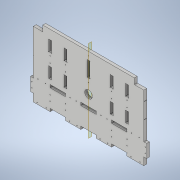
# Autodesk Inventor part: Side_one
Saved by Autodesk Inventor 2020 (Build 240168000, 168)
## iProperties
Created: 2019-12-17
Part Number: Side_one
Material: Generic
Document SubType Name: Modeling
Designer: fabfarm
Density: 1 g/cm^3
Appearance: Default
Author: fabfarm
Autodesk Inventor part; units mm, degrees
ref_plane "YZ Plane" through (0, 0, 0) normal (1, 0, 0) x (0, 1, 0)
ref_plane "XZ Plane" through (0, 0, 0) normal (0, 1, 0) x (-1, 0, 0)
ref_plane "XY Plane" through (0, 0, 0) normal (0, 0, 1) x (1, 0, 0)
sketch "Sketch1" plane through (0, 0, 0) normal (0, 0, 1) x (1, 0, 0)
  line L0 (0, 0) -> (-756, 0)
  line L1 (-756, 0) -> (-756, 464.3)
  line L2 (-756, 464.3) -> (0, 464.3)
  line L3 (0, 464.3) -> (0, 0)
  dimension "d0" = 464.3
  dimension "d1" = 756
  constraints: 8 end point, 2 parallel, 1 horizontal, 1 perpendicular
  measures "d0" distance of L2.end L0.start
  measures "d1" distance of L0.start L0.end
extrude "Extrusion1" add sketch "Sketch1" along normal blind 18.55
sketch "Sketch2" plane through (0, 0, 18.55) normal (0, 0, 1) x (1, 0, 0)
  line L0 (-756, 464.3) -> (-756, 0) projected
  line L1 (-756, 464.3) -> (-737.45, 464.3)
  line L2 (-737.45, 464.3) -> (-737.45, 359.9)
  line L3 (-737.45, 359.9) -> (-756, 359.9)
  line L4 (-756, 359.9) -> (-756, 464.3)
  line L5 (0, 464.3) -> (-756, 464.3) projected
  line L6 (-756, 259.9) -> (-737.45, 259.9)
  line L7 (-737.45, 259.9) -> (-737.45, 134.8)
  line L8 (-737.45, 134.8) -> (-756, 134.8)
  line L9 (-756, 134.8) -> (-756, 259.9)
  point P0 (-756, 359.9)
  point P1 (-756, 134.8)
  dimension "d54" = 18.55
  dimension "d55" = 104.4
  dimension "d86" = 100
  dimension "d87" = 125.1
  constraints: 16 end point, 4 parallel, 2 collinear, 2 horizontal, 2 perpendicular, 2 point on line
  measures "d54" distance of L1.start L1.end
  measures "d55" distance of L1.end L2.end
  measures "d86" distance between parallel lines of L6 L3
  measures "d87" distance of L6.end L7.end
extrude "Extrusion2" cut sketch "Sketch2" against normal blind 18.55
ref_plane "Work Plane1" through (-378, 259.9, 0) normal (-1, 0, 0) x (0, 0, 1)
mirror "Mirror1" about plane through (-378, 259.9, 0) normal (-1, 0, 0) of "Extrusion2"
sketch "Sketch3" plane through (0, 0, 18.55) normal (0, 0, 1) x (1, 0, 0)
  line L0 (0, 464.3) -> (-756, 464.3) projected
  line L1 (-756, 426.35) -> (-676, 426.35)
  line L2 (-676, 426.35) -> (-676, 464.3)
  line L3 (-676, 464.3) -> (-756, 464.3)
  line L4 (-756, 464.3) -> (-756, 426.35)
  point P0 (0, 0)
  point P1 (-18.55, 350)
  point P2 (0, 464.3)
  dimension "d19" = 80
  dimension "d22" = 37.95
  constraints: 8 end point, 2 perpendicular, 1 parallel, 2 other
  measures "d19" distance of L3.end L2.end
  measures "d22" distance of L3.end L1.start
extrude "Extrusion3" cut sketch "Sketch3" against normal blind 18.55
mirror "Mirror2" about plane through (-378, 259.9, 0) normal (-1, 0, 0) of "Extrusion3"
sketch "Sketch4" plane through (0, 0, 18.55) normal (0, 0, 1) x (1, 0, 0)
  line L0 (-628, 134.8) -> (-528, 134.8)
  line L1 (-528, 134.8) -> (-528, 153.35)
  line L2 (-528, 153.35) -> (-628, 153.35)
  line L3 (-628, 153.35) -> (-628, 134.8)
  line L4 (-428, 134.8) -> (-328, 134.8)
  line L5 (-328, 134.8) -> (-328, 153.35)
  line L6 (-328, 153.35) -> (-428, 153.35)
  line L7 (-428, 153.35) -> (-428, 134.8)
  line L8 (-228, 134.8) -> (-128, 134.8)
  line L9 (-128, 134.8) -> (-128, 153.35)
  line L10 (-128, 153.35) -> (-228, 153.35)
  line L11 (-228, 153.35) -> (-228, 134.8)
  line L12 (0, 0) -> (0, 359.9) projected
  line L13 (-756, 359.9) -> (-756, 0) projected
  line L14 (-737.45, 134.8) -> (-756, 134.8) projected
  line L15 (-756, 259.9) -> (-737.45, 259.9) projected
  line L16 (-80, 464.3) -> (-676, 464.3) projected
  line L17 (-378, 464.3) -> (-378, 153.35) construction
  dimension "d59" = 100
  dimension "d60" = 100
  dimension "d61" = 100
  dimension "d62" = 100
  dimension "d63" = 100
  dimension "d66" = 18.55
  constraints: 26 end point, 6 parallel, 5 collinear, 3 horizontal, 3 perpendicular, 2 midpoint, 1 vertical
  measures "d59" distance of L1.end L2.end
  measures "d60" distance of L5.end L6.end
  measures "d61" distance between parallel lines of L1 L7
  measures "d62" distance between parallel lines of L11 L5
  measures "d63" distance of L9.end L10.end
  measures "d66" distance of L2.end L0.start
extrude "Extrusion4" cut sketch "Sketch4" against normal blind 20
sketch "Sketch6" plane through (0, 0, 18.55) normal (0, 0, 1) x (1, 0, 0)
  line L0 (-328, 400.4) -> (-428, 400.4)
  line L1 (-428, 400.4) -> (-428, 425.4)
  line L2 (-428, 425.4) -> (-328, 425.4)
  line L3 (-328, 425.4) -> (-328, 400.4)
  line L4 (-328, 400.4) -> (-428, 425.4) construction
  line L5 (-428, 400.4) -> (-328, 425.4) construction
  line L6 (-378, -92.86) -> (-378, 557.16) projected
  line L7 (-80, 464.3) -> (-676, 464.3) projected
  point P0 (0, 0)
  point P1 (-378, 412.9)
  dimension "d38" = 25
  dimension "d39" = 100
  dimension "d40" = 38.9
  constraints: 12 end point, 2 midpoint, 2 parallel, 1 horizontal, 1 perpendicular, 1 point on line
  measures "d38" distance of L0.end L1.end
  measures "d39" distance of L1.end L2.end
  measures "d40" distance between parallel lines of L7 L2
extrude "Extrusion6" [suppressed]
fillet "Fillet1" [suppressed]
sketch "Sketch7" plane through (0, 0, 18.55) normal (0, 0, 1) x (1, 0, 0)
  line L0 (-637.45, 183.35) -> (-618.9, 183.35)
  line L1 (-618.9, 183.35) -> (-618.9, 253.85)
  line L2 (-618.9, 253.85) -> (-637.45, 253.85)
  line L3 (-637.45, 253.85) -> (-637.45, 183.35)
  line L4 (-537.5, 183.35) -> (-518.95, 183.35)
  line L5 (-518.95, 183.35) -> (-518.95, 253.85)
  line L6 (-518.95, 253.85) -> (-537.5, 253.85)
  line L7 (-537.5, 253.85) -> (-537.5, 183.35)
  line L8 (-676, 464.3) -> (-676, 426.35) projected
  line L9 (-628, 153.35) -> (-528, 153.35) projected
  line L10 (-737.45, 259.9) -> (-737.45, 134.8) projected
  point P0 (0, 0)
  dimension "d44" = 81.4
  dimension "d45" = 18.55
  dimension "d46" = 70.5
  dimension "d72" = 30
  dimension "d194" = 100
  constraints: 16 end point, 4 parallel, 2 horizontal, 2 perpendicular, 2 point on line, 1 collinear
  measures "d44" distance between parallel lines of L7 L1
  measures "d45" distance of L1.end L2.end
  measures "d46" distance of L2.end L0.start
  measures "d72" distance between parallel lines of L9 L0
  measures "d194" distance between parallel lines of L10 L3
extrude "Extrusion7" cut sketch "Sketch7" against normal blind 20
mirror "Mirror3" about plane through (-378, 259.9, 0) normal (-1, 0, 0) of "Extrusion7"
sketch "Esquisse8" plane through (0, 0, 0) normal (0, 0, -1) x (-1, 0, 0)
  line L0 (137.1, 334.35) -> (118.55, 334.35)
  line L1 (118.55, 334.35) -> (118.55, 404.85)
  line L2 (118.55, 404.85) -> (137.1, 404.85)
  line L3 (137.1, 404.85) -> (137.1, 334.35)
  line L4 (218.5, 404.85) -> (237.05, 404.85)
  line L5 (237.05, 404.85) -> (237.05, 334.35)
  line L6 (237.05, 334.35) -> (218.5, 334.35)
  line L7 (218.5, 334.35) -> (218.5, 404.85)
  line L8 (118.55, 183.35) -> (118.55, 253.85) projected
  line L9 (137.1, 253.85) -> (137.1, 183.35) projected
  line L10 (218.5, 183.35) -> (218.5, 253.85) projected
  line L11 (237.05, 253.85) -> (237.05, 183.35) projected
  line L12 (137.1, 253.85) -> (118.55, 253.85) projected
  point P0 (0, 0)
  dimension "d51" = 70.5
  dimension "d90" = 80.5
  constraints: 16 end point, 4 collinear, 4 parallel, 2 horizontal, 2 perpendicular, 2 point on line
  measures "d51" distance of L0.end L1.end
  measures "d90" distance between parallel lines of L0 L12
extrude "Extrusion8" cut sketch "Esquisse8" against normal blind 20
mirror "Symétrie4" about plane through (-378, 259.9, 0) normal (-1, 0, 0) of "Extrusion8"
sketch "Esquisse9" plane through (0, 0, 18.55) normal (0, 0, 1) x (1, 0, 0)
  circle A0 centre (-738.5708, 361.0208) radius 1.585
  circle A1 centre (-738.5708, 135.9208) radius 1.585
  circle A2 centre (-636.3292, 403.7292) radius 1.585
  circle A3 centre (-638.5708, 333.2292) radius 1.585
  circle A4 centre (-738.5708, 258.7792) radius 1.585
  circle A5 centre (-636.3292, 252.7292) radius 1.585
  circle A6 centre (-620.0208, 252.7292) radius 1.585
  circle A7 centre (-620.0208, 184.4708) radius 1.585
  circle A8 centre (-677.1208, 427.4708) radius 1.585
  circle A9 centre (-626.8792, 152.2292) radius 1.585
  circle A10 centre (-426.8792, 152.2292) radius 1.585
  line L0 (-80, 464.3) -> (-676, 464.3) projected
  line L1 (-378, 464.3) -> (-378, 151.8903) construction
  circle A11 centre (-626.8792, 135.9208) radius 1.585
  circle A12 centre (-426.8792, 135.9208) radius 1.585
  line L2 (-737.45, 359.9) -> (-738.5708, 361.0208) construction
  line L3 (-737.45, 426.35) -> (-737.45, 359.9) projected
  line L4 (-737.45, 259.9) -> (-738.5708, 258.7792) construction
  line L5 (-738.5708, 135.9208) -> (-737.45, 134.8) construction
  line L6 (-737.45, 259.9) -> (-737.45, 134.8) projected
  line L7 (-737.45, 426.35) -> (-676, 426.35) projected
  line L8 (-677.1208, 427.4708) -> (-676, 426.35) construction
  line L9 (-637.45, 404.85) -> (-636.3292, 403.7292) construction
  circle A13 centre (-620.0208, 333.2292) radius 1.585
  line L10 (-620.0208, 333.2292) -> (-618.9, 334.35) construction
  line L11 (-637.45, 334.35) -> (-638.5708, 333.2292) construction
  line L12 (-618.9, 334.35) -> (-637.45, 334.35) projected
  line L13 (-620.0208, 184.4708) -> (-618.9, 183.35) construction
  line L14 (-620.0208, 252.7292) -> (-618.9, 253.85) construction
  line L15 (-618.9, 253.85) -> (-618.9, 183.35) projected
  line L16 (-637.45, 183.35) -> (-636.3292, 184.4708) construction
  line L17 (-618.9, 183.35) -> (-637.45, 183.35) projected
  circle A14 centre (-636.3292, 184.4708) radius 1.585
  line L18 (-618.9, 334.35) -> (-618.9, 464.3) projected
  line L19 (-618.9, 411.8699) -> (-537.5, 369.6) construction
  line L20 (-537.5, 334.35) -> (-537.5, 404.85) construction
  line L21 (-578.2, 390.7349) -> (-579.0419, 153.9249) construction
  circle A15 centre (-519.9798, 403.3156) radius 1.585
  circle A16 centre (-518.2397, 332.8014) radius 1.585
  circle A17 centre (-521.0535, 252.3194) radius 1.585
  circle A18 centre (-537.3616, 252.4354) radius 1.585
  circle A19 centre (-537.8469, 184.1786) radius 1.585
  line L22 (-518.8511, 404.4284) -> (-519.9798, 403.3156) construction
  circle A20 centre (-536.7892, 332.9333) radius 1.585
  line L23 (-536.7892, 332.9333) -> (-537.5, 334.35) construction
  line L24 (-519.3524, 333.9301) -> (-518.2397, 332.8014) construction
  line L25 (-537.8469, 184.1786) -> (-538.9756, 183.0658) construction
  line L26 (-537.3616, 252.4354) -> (-538.4743, 253.5641) construction
  line L27 (-520.4261, 182.934) -> (-521.5389, 184.0627) construction
  circle A21 centre (-521.5389, 184.0627) radius 1.585
  line L28 (-537.5, 334.35) -> (-537.5, 404.85)
  line L29 (-537.3508, 411.5799) -> (-619.0492, 369.8899) construction
  line L30 (-528, 134.8) -> (-628, 134.8) construction
  line L31 (-626.8792, 135.9208) -> (-628, 134.8) construction
  line L32 (-628, 153.35) -> (-528, 153.35) construction
  line L33 (-578, 153.35) -> (-578, 134.8) construction
  circle A22 centre (-529.1208, 152.2292) radius 1.585
  circle A23 centre (-529.1208, 135.9208) radius 1.585
  circle A24 centre (-17.4292, 361.0208) radius 1.585
  circle A25 centre (-17.4292, 135.9208) radius 1.585
  circle A26 centre (-136.0858, 403.632) radius 1.585
  line L34 (-119.6708, 403.7292) -> (-136.0858, 403.632) construction
  circle A27 centre (-119.6708, 403.7292) radius 1.585
  circle A28 centre (-117.4292, 333.2292) radius 1.585
  circle A29 centre (-17.4292, 258.7792) radius 1.585
  circle A30 centre (-119.6708, 252.7292) radius 1.585
  circle A31 centre (-135.9792, 252.7292) radius 1.585
  circle A32 centre (-135.9792, 184.4708) radius 1.585
  circle A33 centre (-78.8792, 427.4708) radius 1.585
  circle A34 centre (-129.1208, 152.2292) radius 1.585
  circle A35 centre (-329.1208, 152.2292) radius 1.585
  circle A36 centre (-129.1208, 135.9208) radius 1.585
  circle A37 centre (-329.1208, 135.9208) radius 1.585
  line L35 (-18.55, 359.9) -> (-17.4292, 361.0208) construction
  line L36 (-18.55, 426.35) -> (-18.55, 359.9)
  line L37 (-18.55, 259.9) -> (-17.4292, 258.7792) construction
  line L38 (-17.4292, 135.9208) -> (-18.55, 134.8) construction
  line L39 (-18.55, 259.9) -> (-18.55, 134.8)
  line L40 (-18.55, 426.35) -> (-80, 426.35)
  line L41 (-78.8792, 427.4708) -> (-80, 426.35) construction
  line L42 (-137.1, 404.85) -> (-118.55, 404.85)
  line L43 (-118.55, 404.85) -> (-119.6708, 403.7292) construction
  line L44 (-137.1, 404.85) -> (-136.0858, 403.632) construction
  circle A38 centre (-135.9792, 333.2292) radius 1.585
  line L45 (-135.9792, 333.2292) -> (-137.1, 334.35) construction
  line L46 (-118.55, 334.35) -> (-117.4292, 333.2292) construction
  line L47 (-137.1, 334.35) -> (-118.55, 334.35)
  line L48 (-135.9792, 184.4708) -> (-137.1, 183.35) construction
  line L49 (-135.9792, 252.7292) -> (-137.1, 253.85) construction
  line L50 (-137.1, 253.85) -> (-137.1, 183.35)
  line L51 (-118.55, 183.35) -> (-119.6708, 184.4708) construction
  line L52 (-137.1, 183.35) -> (-118.55, 183.35)
  circle A39 centre (-119.6708, 184.4708) radius 1.585
  line L53 (-137.1, 334.35) -> (-137.1, 404.85)
  line L54 (-137.1, 411.8699) -> (-218.5, 369.6) construction
  line L55 (-218.5, 334.35) -> (-218.5, 404.85) construction
  line L56 (-177.8, 390.7349) -> (-176.9581, 153.9249) construction
  circle A40 centre (-218.6384, 252.4354) radius 1.585
  circle A41 centre (-218.1531, 184.1786) radius 1.585
  circle A42 centre (-219.3052, 403.2183) radius 1.8195
  circle A43 centre (-234.9465, 252.3194) radius 1.585
  line L57 (-218.1531, 184.1786) -> (-217.0244, 183.0658) construction
  line L58 (-218.6384, 252.4354) -> (-217.5257, 253.5641) construction
  line L59 (-235.5739, 182.934) -> (-234.4611, 184.0627) construction
  circle A44 centre (-234.4611, 184.0627) radius 1.585
  line L60 (-236.0202, 403.3156) -> (-219.3052, 403.2183) construction
  circle A45 centre (-237.7603, 332.8014) radius 1.585
  line L61 (-236.6476, 333.9301) -> (-237.7603, 332.8014) construction
  circle A46 centre (-219.2108, 332.9333) radius 1.585
  line L62 (-218.6492, 411.5799) -> (-136.9508, 369.8899) construction
  line L63 (-218.5, 334.35) -> (-218.5, 404.85)
  line L64 (-219.2108, 332.9333) -> (-218.5, 334.35) construction
  circle A47 centre (-236.0202, 403.3156) radius 1.585
  line L65 (-237.1489, 404.4284) -> (-236.0202, 403.3156) construction
  line L66 (-218.5, 404.85) -> (-219.3052, 403.2183) construction
  line L67 (-228, 134.8) -> (-128, 134.8) construction
  line L68 (-129.1208, 135.9208) -> (-128, 134.8) construction
  line L69 (-128, 153.35) -> (-228, 153.35) construction
  line L70 (-178, 153.35) -> (-178, 134.8) construction
  circle A48 centre (-226.8792, 152.2292) radius 1.585
  circle A49 centre (-226.8792, 135.9208) radius 1.585
  line L71 (-637.45, 404.85) -> (-618.9, 404.85) projected
  circle A50 centre (-620.0208, 403.7292) radius 1.585
  line L72 (-618.9, 404.85) -> (-620.0208, 403.7292) construction
  circle A51 centre (-536.2879, 403.4315) radius 1.585
  point P0 (-518.95, 183.35)
  point P1 (-328, 153.35)
  point P2 (-518.95, 404.85)
  point P3 (-428, 134.8)
  point P4 (-228, 153.35)
  point P5 (-237.05, 183.35)
  point P6 (-237.05, 404.85)
  point P7 (-128, 153.35)
  point P8 (-328, 134.8)
  dimension "d69" = 3.17
  dimension "d115" = 45
  dimension "d117" = 45
  dimension "d118" = 45
  dimension "d119" = 45
  dimension "d123" = 45
  dimension "d129" = 45
  dimension "d130" = 45
  dimension "d131" = 45
  dimension "d132" = 45
  dimension "d143" = 45
  dimension "d144" = 45
  constraints: 116 end point, 86 symmetric about line, 20 vertical, 14 coincident, 11 centre point, 5 horizontal alignment, 4 midpoint, 3 vertical alignment, 154 other
  measures "d115" angle of L3 L2
  measures "d117" angle of L6 L5
  measures "d118" angle of L6 L4
  measures "d119" angle of L7 L8
  measures "d123" angle of L12 L11
  measures "d129" angle of L15 L14
  measures "d130" angle of L15 L13
  measures "d131" angle of L17 L16
  measures "d132" angle of L30 L31
  measures "d143" angle of L9 L71
  measures "d144" angle to the sketch x axis of L72
extrude "Extrusion9" cut sketch "Esquisse9" against normal blind 20
sketch "Esquisse11" plane through (0, 0, 18.55) normal (0, 0, 1) x (1, 0, 0)
  circle A0 centre (-746.725, 329.9) radius 2.25
  circle A1 centre (-746.725, 289.9) radius 2.25
  circle A2 centre (-628.175, 314.35) radius 2.25
  circle A3 centre (-628.175, 273.85) radius 2.25
  circle A4 centre (-528.225, 314.35) radius 2.25
  circle A5 centre (-528.225, 273.85) radius 2.25
  line L0 (-618.9, 334.35) -> (-637.45, 334.35) projected
  line L1 (-628.175, 334.35) -> (-628.175, 253.85) construction
  line L2 (-637.45, 253.85) -> (-618.9, 253.85) projected
  line L3 (-518.95, 334.35) -> (-537.5, 334.35) projected
  line L4 (-528.225, 334.35) -> (-528.225, 253.85) construction
  line L5 (-537.5, 253.85) -> (-518.95, 253.85) projected
  line L6 (-737.45, 359.9) -> (-756, 359.9) projected
  line L7 (-80, 464.3) -> (-676, 464.3) projected
  line L8 (-378, 464.3) -> (-378, 153.35) construction
  line L9 (-428, 153.35) -> (-328, 153.35) projected
  circle A6 centre (-9.275, 329.9) radius 2.25
  circle A7 centre (-9.275, 289.9) radius 2.25
  circle A8 centre (-127.825, 314.35) radius 2.25
  circle A9 centre (-127.825, 273.85) radius 2.25
  circle A10 centre (-227.775, 314.35) radius 2.25
  circle A11 centre (-227.775, 273.85) radius 2.25
  line L10 (-127.825, 334.35) -> (-127.825, 253.85) construction
  line L11 (-120.7915, 253.85) -> (-134.8585, 253.85)
  line L12 (-282.265, 334.65) -> (-266.585, 334.65)
  line L13 (-227.775, 334.35) -> (-227.775, 253.85) construction
  line L14 (-266.585, 253.65) -> (-282.265, 253.65)
  line L15 (-16.3085, 359.9) -> (0, 359.9)
  line L16 (-756, 259.9) -> (-737.45, 259.9) projected
  line L17 (-746.725, 359.9) -> (-746.725, 259.9) construction
  point P0 (-573.5723, 199.8)
  point P1 (-692.3085, 334.35)
  point P2 (-635.2085, 253.85)
  point P3 (-621.1415, 253.85)
  point P4 (-473.735, 334.65)
  point P5 (-489.415, 334.65)
  point P6 (-489.415, 253.65)
  point P7 (-473.735, 253.65)
  point P8 (-739.6915, 359.9)
  point P9 (-425.7585, 153.35)
  point P10 (-277.485, 153.35)
  point P11 (-266.585, 253.65)
  point P12 (-739.6915, 259.9)
  dimension "d76" = 4.5
  dimension "d79" = 30
  dimension "d80" = 20
  dimension "d81" = 20
  dimension "d82" = 20
  dimension "d83" = 20
  dimension "d91" = 30
  constraints: 18 symmetric about line, 16 end point, 12 centre point, 10 point on line, 5 equal radius, 5 midpoint, 18 other
  measures "d76" diameter of A0
  measures "d79" distance from line of L6 A0.centre
  measures "d80" distance from line of L2 A3.centre
  measures "d91" distance from line of A1.centre L16
extrude "Extrusion10" cut sketch "Esquisse11" against normal blind 20
sketch "Esquisse12" plane through (0, 0, 18.55) normal (0, 0, 1) x (1, 0, 0)
  line L0 (-756, 0) -> (0, 0) projected
  line L1 (-628, 0) -> (-528, 0)
  line L2 (-528, 0) -> (-528, 18.55)
  line L3 (-528, 18.55) -> (-628, 18.55)
  line L4 (-628, 18.55) -> (-628, 0)
  line L5 (-428, 0) -> (-328, 0)
  line L6 (-328, 0) -> (-328, 18.55)
  line L7 (-328, 18.55) -> (-428, 18.55)
  line L8 (-428, 18.55) -> (-428, 0)
  line L9 (-228, 0) -> (-128, 0)
  line L10 (-128, 0) -> (-128, 18.55)
  line L11 (-128, 18.55) -> (-228, 18.55)
  line L12 (-228, 18.55) -> (-228, 0)
  line L13 (-528, 153.35) -> (-528, 134.8) projected
  line L14 (-628, 134.8) -> (-628, 153.35) projected
  line L15 (-428, 134.8) -> (-428, 153.35) projected
  line L16 (-328, 153.35) -> (-328, 134.8) projected
  line L17 (-228, 134.8) -> (-228, 153.35) projected
  line L18 (-128, 153.35) -> (-128, 134.8) projected
  point P0 (-475.9, 151.865)
  point P1 (-475.9, 136.385)
  point P2 (-628, 137.0415)
  point P3 (-628, 151.1085)
  point P4 (-428, 137.0415)
  point P5 (-428, 151.1085)
  point P6 (-275.9, 151.865)
  point P7 (-275.9, 136.385)
  point P8 (-176.1, 136.385)
  point P9 (-176.1, 151.865)
  point P10 (-75.9, 151.865)
  point P11 (-75.9, 136.385)
  point P12 (-128, 0)
  point P13 (-528, 0)
  point P14 (-328, 0)
  dimension "d92" = 18.55
  constraints: 24 end point, 6 parallel, 4 point on line, 4 vertical, 3 collinear, 3 horizontal, 3 perpendicular, 4 other
  measures "d92" distance of L3.end L1.start
extrude "Extrusion11" cut sketch "Esquisse12" against normal blind 20
sketch "Esquisse13" plane through (0, 0, 18.55) normal (0, 0, 1) x (1, 0, 0)
  circle A0 centre (-626.8686, 17.4186) radius 1.6
  line L0 (-628, 0) -> (-628, 18.55) construction
  line L1 (-628, 18.55) -> (-626.8686, 17.4186) construction
  line L2 (-628, 18.55) -> (-528, 18.55) projected
  circle A1 centre (-529.1314, 17.4186) radius 1.6
  circle A2 centre (-426.8686, 17.4186) radius 1.6
  line L3 (-378, 18.55) -> (-378, 134.8) construction
  line L4 (-328, 134.8) -> (-428, 134.8) projected
  line L5 (-428, 18.55) -> (-328, 18.55) projected
  circle A3 centre (-129.1314, 17.4186) radius 1.6
  line L6 (-128, 0) -> (-128, 18.55) construction
  line L7 (-128, 18.55) -> (-129.1314, 17.4186) construction
  line L8 (-128, 18.55) -> (-228, 18.55) construction
  circle A4 centre (-226.8686, 17.4186) radius 1.6
  circle A5 centre (-329.1314, 17.4186) radius 1.6
  point P0 (0, 0)
  point P1 (-228, 18.55)
  point P2 (-128, 18.55)
  point P3 (-330.2415, 134.8)
  point P4 (-425.7585, 134.8)
  point P5 (-225.7373, 18.55)
  point P6 (-530.2627, 18.55)
  dimension "d95" = 3.2
  dimension "d133" = 45
  constraints: 10 end point, 6 symmetric about line, 4 vertical, 2 horizontal alignment, 2 midpoint, 18 other
  measures "d133" angle of L2 L1
extrude "Extrusion12" cut sketch "Esquisse13" against normal blind 20
sketch "Esquisse14" plane through (0, 0, 18.55) normal (0, 0, 1) x (1, 0, 0)
  circle A0 centre (-628.175, 94.8) radius 2.25
  circle A1 centre (-628.175, 58.55) radius 2.25
  circle A2 centre (-528.225, 94.8) radius 2.25
  circle A3 centre (-528.225, 58.55) radius 2.25
  line L0 (-618.9, 183.35) -> (-637.45, 183.35) projected
  line L1 (-628.175, 183.35) -> (-628.175, 0) construction
  line L2 (-756, 0) -> (-628, 0) projected
  line L3 (-518.95, 183.35) -> (-537.5, 183.35) projected
  line L4 (-528.225, 183.35) -> (-528.225, -0.1) construction
  line L5 (-625.7373, 18.55) -> (-528, 18.55) projected
  line L6 (-528, 134.8) -> (-628, 134.8) projected
  line L7 (-428, 18.55) -> (-328, 18.55) projected
  line L8 (-378, 18.55) -> (-378, 134.8) construction
  line L9 (-328, 134.8) -> (-428, 134.8) projected
  circle A4 centre (-127.825, 94.8) radius 2.25
  circle A5 centre (-127.825, 58.55) radius 2.25
  circle A6 centre (-227.775, 94.8) radius 2.25
  circle A7 centre (-227.775, 58.55) radius 2.25
  point P0 (0, 0)
  point P1 (-477.5, 18.55)
  point P2 (-477.485, 134.8)
  point P3 (-625.7585, 134.8)
  point P4 (-374.5, 18.55)
  point P5 (-277.5, 18.55)
  point P6 (-277.485, 134.8)
  point P7 (-425.7585, 134.8)
  dimension "d98" = 4.5
  dimension "d99" = 40
  dimension "d100" = 40
  dimension "d101" = 40
  dimension "d103" = 40
  constraints: 8 centre point, 6 end point, 5 point on line, 4 midpoint, 4 symmetric about line, 3 equal radius, 2 vertical, 4 other
  measures "d98" diameter of A0
  measures "d99" distance from line of L5 A3.centre
  measures "d100" distance from line of L6 A2.centre
  measures "d101" distance from line of L6 A0.centre
  measures "d103" distance from line of L5 A1.centre
extrude "Extrusion13" cut sketch "Esquisse14" against normal blind 20
sketch "Esquisse16" plane through (0, 0, 18.55) normal (0, 0, 1) x (1, 0, 0)
  line L0 (0, 0) -> (0, 134.8) projected
  line L1 (-128, 0) -> (0, 0) projected
  line L2 (0, 50) -> (-18.55, 50)
  line L3 (-18.55, 50) -> (-18.55, 0)
  line L4 (-18.55, 0) -> (0, 0)
  line L5 (0, 0) -> (0, 50)
  line L6 (-18.55, 134.8) -> (-18.55, 259.9) projected
  line L7 (0, 134.8) -> (-18.55, 134.8) projected
  line L8 (-756, 0) -> (-628, 0) projected
  line L9 (-756, 50) -> (-737.45, 50)
  line L10 (-737.45, 50) -> (-737.45, 0)
  line L11 (-737.45, 0) -> (-756, 0)
  line L12 (-756, 0) -> (-756, 50)
  line L13 (-737.45, 259.9) -> (-737.45, 134.8) projected
  line L14 (-756, 134.8) -> (-756, 0) projected
  point P0 (-18.55, 136.385)
  point P1 (-18.55, 258.315)
  point P2 (-16.965, 134.8)
  dimension "d110" = 50
  dimension "d111" = 84.8
  constraints: 16 end point, 4 collinear, 4 parallel, 3 point on line, 2 horizontal, 2 perpendicular
  measures "d110" distance of L2.end L3.end
  measures "d111" distance between parallel lines of L7 L2
extrude "Extrusion15" cut sketch "Esquisse16" against normal blind 60
sketch "Esquisse18" plane through (0, 0, 18.55) normal (0, 0, 1) x (1, 0, 0)
  line L0 (-737.45, 50) -> (-737.45, 0) projected
  circle A0 centre (-738.5814, 48.8686) radius 1.6
  circle A1 centre (-17.4186, 48.8686) radius 1.6
  line L1 (-18.55, 50) -> (0, 50) construction
  line L2 (-18.55, 50) -> (-17.4186, 48.8686) construction
  line L3 (-18.55, 0) -> (-18.55, 50) construction
  point P0 (0, 0)
  dimension "d136" = 3.2
  dimension "d135" = 45
  constraints: 2 end point, 1 horizontal alignment, 6 other
  measures "d135" angle of L3 L2
extrude "Extrusion16" cut sketch "Esquisse18" against normal blind 20
sketch "Esquisse17" plane through (0, 0, 18.55) normal (0, 0, 1) x (1, 0, 0)
  circle A0 centre (-8.9415, 109.8) radius 2.25
  circle A1 centre (-8.9415, 75) radius 2.25
  circle A2 centre (-747.5228, 109.8) radius 2.25
  circle A3 centre (-747.5228, 75) radius 2.25
  line L0 (-756, 134.8) -> (-737.45, 134.8) projected
  line L1 (-746.725, 134.8) -> (-747.8564, 50) construction
  line L2 (-739.7127, 50) -> (-756, 50) projected
  line L3 (-18.55, 134.8) -> (0, 134.8) construction
  line L4 (-9.275, 134.8) -> (-8.1436, 50) construction
  line L5 (-16.2873, 50) -> (0, 50) construction
  point P0 (0, 0)
  point P1 (-739.6915, 134.8)
  point P2 (-16.3085, 134.8)
  dimension "d134" = 4.5
  dimension "d139" = 25
  dimension "d140" = 25
  constraints: 4 centre point, 4 end point, 4 midpoint, 3 equal radius, 2 horizontal alignment, 2 point on line, 2 vertical alignment
  measures "d134" diameter of A2
  measures "d139" distance from line of L0 A2.centre
  measures "d140" distance from line of A3.centre L2
extrude "Extrusion17" cut sketch "Esquisse17" against normal blind 20
sketch "Esquisse19" plane through (0, 0, 18.55) normal (0, 0, 1) x (1, 0, 0)
  line L0 (-518.95, 402.1107) -> (-518.95, 404.5204) projected
  line L1 (-368.725, 314.3) -> (-387.275, 314.3)
  line L2 (-387.275, 314.3) -> (-387.275, 414.3)
  line L3 (-387.275, 414.3) -> (-368.725, 414.3)
  line L4 (-368.725, 414.3) -> (-368.725, 314.3)
  line L5 (-80, 464.3) -> (-676, 464.3) projected
  line L6 (-378, 464.3) -> (-378, 414.3) construction
  point P0 (0, 0)
  point P1 (-576.05, 336.5915)
  dimension "d169" = 100
  dimension "d170" = 18.55
  dimension "d171" = 50
  constraints: 10 end point, 2 midpoint, 2 parallel, 1 horizontal, 1 perpendicular, 1 vertical, 1 other
  measures "d169" distance of L3.end L1.start
  measures "d170" distance of L1.start L1.end
  measures "d171" distance between parallel lines of L5 L3
extrude "Extrusion18" cut sketch "Esquisse19" against normal blind 18.55
sketch "Esquisse20" plane through (0, 0, 18.55) normal (0, 0, 1) x (1, 0, 0)
  line L0 (0, 259.9) -> (-18.55, 259.9)
  line L1 (-18.55, 259.9) -> (-18.55, 359.9)
  line L2 (-18.55, 359.9) -> (0, 359.9)
  line L3 (0, 359.9) -> (0, 259.9)
  line L4 (-737.45, 137.0415) -> (-737.45, 257.6585) projected
  line L5 (-737.45, 259.9) -> (-756, 259.9)
  line L6 (-756, 259.9) -> (-756, 359.9)
  line L7 (-756, 359.9) -> (-737.45, 359.9)
  line L8 (-737.45, 359.9) -> (-737.45, 259.9)
  line L9 (0, 359.9) -> (-18.55, 359.9) projected
  line L10 (-756, 359.9) -> (-756, 259.9) projected
  line L11 (-18.55, 359.9) -> (-18.55, 426.35) projected
  point P0 (0, 0)
  point P1 (-16.3085, 359.9)
  point P2 (-18.55, 362.1415)
  constraints: 16 end point, 5 collinear, 4 parallel, 2 horizontal, 2 perpendicular, 1 point on line
extrude "Extrusion19" cut sketch "Esquisse20" against normal blind 18.55
sketch "Esquisse21" plane through (0, 0, 18.55) normal (0, 0, 1) x (1, 0, 0)
  circle A0 centre (-378, 223.35) radius 25
  line L0 (-425.7585, 153.35) -> (-328, 153.35) projected
  line L1 (-378, 223.35) -> (-378, 464.3) construction
  line L2 (-80, 464.3) -> (-676, 464.3) projected
  point P0 (0, 0)
  dimension "d157" = 50
  dimension "d191" = 70
  constraints: 2 end point, 1 centre point, 1 midpoint, 1 vertical
  measures "d157" diameter of A0
  measures "d191" distance from line of L0 L1.start
extrude "Extrusion20" cut sketch "Esquisse21" against normal blind 18.55
sketch "Esquisse22" plane through (0, 0, 18.55) normal (0, 0, 1) x (1, 0, 0)
  circle A0 centre (-303, 9) radius 2.25
  circle A1 centre (-253, 9) radius 2.25
  circle A2 centre (-503, 9) radius 2.25
  circle A3 centre (-453, 9) radius 2.25
  line L0 (-528, 16.2873) -> (-528, 0) projected
  line L1 (-428, 0) -> (-428, 16.2873) projected
  line L2 (-328, 16.2873) -> (-328, 0) projected
  line L3 (-228, 0) -> (-228, 16.2873) projected
  line L4 (-328, 0) -> (-228, 0) projected
  circle A4 centre (-653, 9) radius 2.25
  circle A5 centre (-712.45, 9) radius 2.25
  line L5 (-628, 0) -> (-628, 16.2873) projected
  line L6 (-737.45, 47.7373) -> (-737.45, 0) projected
  circle A6 centre (-103, 9) radius 2.25
  circle A7 centre (-43.55, 9) radius 2.25
  line L7 (-128, 16.2873) -> (-128, 0) projected
  line L8 (-18.55, 0) -> (-18.55, 47.7373) projected
  point P0 (0, 0)
  dimension "d161" = 25
  dimension "d162" = 25
  dimension "d163" = 25
  dimension "d164" = 25
  dimension "d165" = 4.5
  dimension "d166" = 9
  dimension "d195" = 25
  dimension "d196" = 25
  dimension "d197" = 25
  dimension "d198" = 25
  constraints: 8 centre point, 7 equal radius, 7 horizontal alignment
  measures "d161" distance from line of L0 A2.centre
  measures "d162" distance from line of L1 A3.centre
  measures "d163" distance from line of L2 A0.centre
  measures "d164" distance from line of L3 A1.centre
  measures "d165" diameter of A0
  measures "d166" distance from line of L4 A0.centre
  measures "d195" distance from line of L5 A4.centre
  measures "d196" distance from line of L6 A5.centre
  measures "d197" distance from line of A6.centre L7
  measures "d198" distance from line of L8 A7.centre
extrude "Extrusion21" cut sketch "Esquisse22" against normal blind 20
sketch "Esquisse24" plane through (0, 0, 18.55) normal (0, 0, 1) x (1, 0, 0)
  circle A0 centre (-386.1436, 413.1686) radius 1.6
  circle A1 centre (-369.8564, 413.1686) radius 1.6
  circle A2 centre (-386.1436, 315.4314) radius 1.6
  line L0 (-368.725, 414.3) -> (-368.725, 314.3) projected
  circle A3 centre (-369.8564, 315.4314) radius 1.6
  line L1 (-387.275, 314.3) -> (-387.275, 414.3) projected
  line L2 (-387.275, 414.3) -> (-386.1436, 413.1686) construction
  circle A4 centre (-378, 289.3) radius 2.25
  line L3 (-387.275, 314.3) -> (-368.725, 314.3) projected
  line L4 (-378, 314.3) -> (-378, 289.3) construction
  circle A5 centre (-377.95, 439.3) radius 2.25
  line L5 (-387.275, 414.3) -> (-368.725, 414.3) projected
  point P0 (0, 0)
  dimension "d173" = 3.2
  dimension "d174" = 45
  dimension "d175" = 4.5
  dimension "d176" = 25
  dimension "d177" = 25
  dimension "d178" = 4.5
  dimension "d179" = 9.325
  constraints: 4 end point, 3 centre point, 2 horizontal alignment, 2 vertical alignment, 1 midpoint, 1 vertical, 12 other
  measures "d174" angle of L1 L2
  measures "d175" diameter of A4
  measures "d176" distance of L4.start L4.end
  measures "d177" distance from line of L5 A5.centre
  measures "d178" diameter of A5
  measures "d179" distance from line of L1 A5.centre
extrude "Extrusion22" cut sketch "Esquisse24" against normal blind 18.55 contours A0 L1 L5 | L5 A0 | A0 L1 | L5 L0 A1 | A1 L5 | L1 A2 | A2 L3 L1 | A1 L0 | L3 A2 | A3 L0 | L0 L3 A3 | A3 L3 | A4 | A5
sketch "Esquisse25" plane through (0, 0, 18.55) normal (0, 0, 1) x (1, 0, 0)
  line L0 (-528, 151.1085) -> (-528, 137.0415) projected
  line L1 (-528, 144.075) -> (-428, 144.075) construction
  line L2 (-428, 137.0415) -> (-428, 151.1085) projected
  circle A0 centre (-498, 144.075) radius 2.25
  circle A1 centre (-458, 144.075) radius 2.25
  circle A2 centre (-298, 144.075) radius 2.25
  circle A3 centre (-258, 144.075) radius 2.25
  circle A4 centre (-98, 144.075) radius 2.25
  circle A5 centre (-658, 144.075) radius 2.25
  line L3 (-628, 137.0415) -> (-628, 151.1085) projected
  line L4 (-128, 153.35) -> (-128, 134.8) projected
  line L5 (-228, 134.8) -> (-228, 153.35) projected
  line L6 (-328, 153.35) -> (-328, 134.8) projected
  circle A6 centre (-707.45, 144.075) radius 2.25
  circle A7 centre (-48.55, 144.075) radius 2.25
  line L7 (-737.45, 257.6585) -> (-737.45, 137.0415) projected
  line L8 (-18.55, 137.0415) -> (-18.55, 257.6585) projected
  point P0 (0, 0)
  point P1 (-128, 151.1085)
  point P2 (-128, 137.0415)
  point P3 (-228, 137.0415)
  point P4 (-228, 151.1085)
  point P5 (-328, 151.1085)
  point P6 (-328, 137.0415)
  dimension "d182" = 30
  dimension "d183" = 30
  dimension "d184" = 30
  dimension "d185" = 30
  dimension "d186" = 30
  dimension "d187" = 30
  dimension "d188" = 4.5
  dimension "d192" = 30
  dimension "d193" = 30
  constraints: 8 centre point, 7 equal radius, 7 horizontal alignment, 2 end point, 2 midpoint, 2 point on line, 1 horizontal
  measures "d182" distance from line of L3 A5.centre
  measures "d183" distance from line of L4 A4.centre
  measures "d184" distance from line of L5 A3.centre
  measures "d185" distance from line of L6 A2.centre
  measures "d186" horizontal distance of L2.start A1.centre
  measures "d187" distance from line of L0 A0.centre
  measures "d188" diameter of A1
  measures "d192" distance from line of A6.centre L7
  measures "d193" distance from line of L8 A7.centre
extrude "Extrusion23" cut sketch "Esquisse25" against normal blind 30
body "Solid1"
